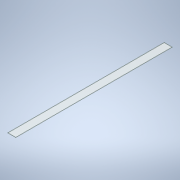
# Autodesk Inventor part: Tapa para soporte Led-2
Saved by Autodesk Inventor 2020 (Build 240168000, 168)
## iProperties
Created: 2020-11-14
Part Number: Tapa para soporte Led-2
Material: Genérico
Document SubType Name: Modeling
Designer: Pipi
Density: 1 g/cm^3
Appearance: Claro
Author: Pipi
Autodesk Inventor part; units mm, degrees
ref_plane "YZ Plane" through (0, 0, 0) normal (1, 0, 0) x (0, 1, 0)
ref_plane "XZ Plane" through (0, 0, 0) normal (0, 1, 0) x (-1, 0, 0)
ref_plane "XY Plane" through (0, 0, 0) normal (0, 0, 1) x (1, 0, 0)
sketch "Boceto1" plane through (0, 0, 0) normal (0, 1, 0) x (-1, 0, 0)
  line L0 (9.2786, 369.1337) -> (-8.7214, 369.1337)
  line L1 (-8.7214, 369.1337) -> (-8.7214, 15.1337)
  line L2 (-8.7214, 15.1337) -> (9.2786, 15.1337)
  line L3 (9.2786, 15.1337) -> (9.2786, 369.1337)
  point P0 (0, 0)
  dimension "d0" = 18
  dimension "d1" = 354
  constraints: 8 end point, 2 parallel, 1 horizontal, 1 perpendicular
  measures "d0" distance of L2.end L1.end
  measures "d1" distance of L0.end L1.end
extrude "Extrusión1" add sketch "Boceto1" along normal blind 1
